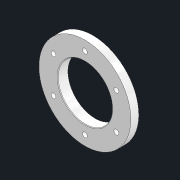
# Autodesk Inventor part: base12
Saved by Autodesk Inventor 2021 (Build 250183000, 183)
## iProperties
Created: 2021-07-25
Part Number: base12
Material: ABS プラスチック
Document SubType Name: Modeling
Designer: yuto6
Density: 1.06 g/cm^3
Appearance: 滑らか - 白
Author: yuto6
Autodesk Inventor part; units mm, degrees
ref_plane "YZ Plane" through (0, 0, 0) normal (1, 0, 0) x (0, 1, 0)
ref_plane "XZ Plane" through (0, 0, 0) normal (0, 1, 0) x (-1, 0, 0)
ref_plane "XY Plane" through (0, 0, 0) normal (0, 0, 1) x (1, 0, 0)
sketch "スケッチ2" plane through (0, 0, 0) normal (1, 0, 0) x (0, 1, 0)
  line L0 (24, 0) -> (24, -9)
  line L1 (40.5, 0) -> (40.5, -7)
  line L2 (40.5, 0) -> (24, 0)
  line L3 (24, 0) -> (59, 0)
  line L4 (24, -9) -> (28, -9)
  line L5 (0, -10.8) -> (0, 1.8) projected
  line L6 (28, -9) -> (28, -7)
  line L7 (28, -7) -> (40.5, -7)
  point P0 (0, 0)
  dimension "d40" = 24
  dimension "d41" = 7
  dimension "d42" = 40.5
  dimension "d43" = 28
  dimension "d44" = 2
  constraints: 14 end point, 3 horizontal, 3 perpendicular, 1 horizontal alignment, 1 vertical
  measures "d40" distance from line of point (0, 0) L0
  measures "d41" distance of L1.end L1.start
  measures "d42" distance from line of point (0, 0) L1
  measures "d43" distance between parallel lines of L5 L6
  measures "d44" distance of L4.end L6.end
revolve "回転1" add sketch "スケッチ2" angle 360 about axis through (0, 0, -10) along (0, 0, 1)
sketch "スケッチ4" plane through (0, 0, 0) normal (0, 0, 1) x (1, 0, 0)
  point P0 (0, 0)
  point P1 (0, 32)
  point P2 (-27.7128, 16)
  point P3 (-27.7128, -16)
  point P4 (0, -32)
  point P5 (27.7128, -16)
  point P6 (27.7128, 16)
  dimension "d11" = 32
  dimension "d14" = 360
  constraints: 7 other
  measures "d11" distance of point (0, 0) point (0, 32)
hole "穴1" at (0, 32, 0) at (-27.7128, 16, 0) at (-27.7128, -16, 0) at (0, -32, 0) at (27.7128, -16, 0) at (27.7128, 16, 0) direction (0, 0, -1) diameter 4.3 end through all clearance for "Socket Head Cap Screw" size "M4" standard "Ansi Metric M Profile"
chamfer "面取り3" distance 0.5 angle 45 1 edges at (0, -28, -9)
chamfer "面取り4" distance 0.5 angle 45 1 edges at (0, -24, 0)
